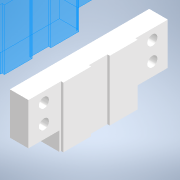
# Autodesk Inventor part: YCarriageBackHolder
Saved by Autodesk Inventor 2020 (Build 240168000, 168)
## iProperties
Created: 2022-04-26
Part Number: YCarriageBackHolder
Material: Tworzywo sztuczne ABS
Document SubType Name: Modeling
Designer: mikoma
Density: 1.06 g/cm^3
Appearance: Gładki — biały
Mass: 37.5008 g
Surface Area: 105.956 cm^2
Volume: 35.3781 cm^3
Author: mikoma
Autodesk Inventor part; units mm, degrees
ref_plane "YZ Plane" through (0, 0, 0) normal (1, 0, 0) x (0, 1, 0)
ref_plane "XZ Plane" through (0, 0, 0) normal (0, 1, 0) x (-1, 0, 0)
ref_plane "XY Plane" through (0, 0, 0) normal (0, 0, 1) x (1, 0, 0)
sketch "Szkic1" plane through (0, 0, 0) normal (0, 1, 0) x (-1, 0, 0)
  line L0 (12, 45) -> (0, 45)
  line L1 (0, 45) -> (0, -45)
  line L2 (0, -45) -> (12, -45)
  line L3 (12, -45) -> (12, 45)
  line L4 (0, 24) -> (-1.5, 24)
  line L5 (-1.5, 24) -> (-1.5, 6)
  line L6 (-1.5, 6) -> (0, 6)
  line L7 (0, 6) -> (0, 24)
  line L8 (0, -6) -> (-1.5, -6)
  line L9 (-1.5, -6) -> (-1.5, -24)
  line L10 (-1.5, -24) -> (0, -24)
  line L11 (0, -24) -> (0, -6)
  point P0 (0, 0)
  point P1 (0, -24)
  point P2 (0, 6)
  dimension "d0" = 90
  dimension "d1" = 12
  dimension "d2" = 45
  dimension "d3" = 21
  dimension "d4" = 18
  dimension "d5" = 1.5
  dimension "d6" = 21
  dimension "d7" = 18
  constraints: 24 end point, 6 parallel, 3 horizontal, 3 perpendicular, 2 point on line, 1 midpoint, 1 vertical alignment
  measures "d0" distance of L2.end L0.start
  measures "d1" distance of L1.end L2.end
  measures "d2" distance from line of L2 point (0, 0)
  measures "d3" distance between parallel lines of L0 L4
  measures "d4" distance between parallel lines of L4 L6
  measures "d5" distance from line of L0.end L5
  measures "d6" distance from line of L2 L9.end
  measures "d7" distance of L8.end L9.end
extrude "Wyciągnięcie proste1" add sketch "Szkic1" along normal blind 39
sketch "Szkic2" plane through (-12, 0, -45) normal (-1, 0, 0) x (0, 0, 1)
  circle A0 centre (10, 32.5) radius 3.25
  circle A1 centre (10, 20.5) radius 3.25
  circle A2 centre (80, 32.5) radius 3.25
  circle A3 centre (80, 20.5) radius 3.25
  line L0 (0, 39) -> (90, 39) projected
  line L1 (0, 0) -> (0, 39) projected
  line L2 (90, 0) -> (90, 39) projected
  line L3 (0, 0) -> (20, 0)
  line L4 (20, 0) -> (20, 12)
  line L5 (20, 12) -> (0, 12)
  line L6 (0, 12) -> (0, 0)
  line L7 (0, 0) -> (90, 0) projected
  line L8 (90, 0) -> (70, 0)
  line L9 (70, 0) -> (70, 12)
  line L10 (70, 12) -> (90, 12)
  line L11 (90, 12) -> (90, 0)
  line L12 (13.0311, 37.75) -> (16.0622, 32.5)
  line L13 (16.0622, 32.5) -> (13.0311, 27.25)
  line L14 (13.0311, 27.25) -> (6.9689, 27.25)
  line L15 (6.9689, 27.25) -> (3.9378, 32.5)
  line L16 (3.9378, 32.5) -> (6.9689, 37.75)
  line L17 (6.9689, 37.75) -> (13.0311, 37.75)
  line L18 (13.0311, 25.75) -> (16.0622, 20.5)
  line L19 (16.0622, 20.5) -> (13.0311, 15.25)
  line L20 (13.0311, 15.25) -> (6.9689, 15.25)
  line L21 (6.9689, 15.25) -> (3.9378, 20.5)
  line L22 (3.9378, 20.5) -> (6.9689, 25.75)
  line L23 (6.9689, 25.75) -> (13.0311, 25.75)
  line L24 (76.9689, 25.75) -> (83.0311, 25.75)
  line L25 (83.0311, 25.75) -> (86.0622, 20.5)
  line L26 (86.0622, 20.5) -> (83.0311, 15.25)
  line L27 (83.0311, 15.25) -> (76.9689, 15.25)
  line L28 (76.9689, 15.25) -> (73.9378, 20.5)
  line L29 (73.9378, 20.5) -> (76.9689, 25.75)
  line L30 (76.9689, 37.75) -> (83.0311, 37.75)
  line L31 (83.0311, 37.75) -> (86.0622, 32.5)
  line L32 (86.0622, 32.5) -> (83.0311, 27.25)
  line L33 (83.0311, 27.25) -> (76.9689, 27.25)
  line L34 (76.9689, 27.25) -> (73.9378, 32.5)
  line L35 (73.9378, 32.5) -> (76.9689, 37.75)
  point P0 (45, 0)
  point P1 (0, 12)
  dimension "d10" = 6.5
  dimension "d11" = 6.5
  dimension "d12" = 10
  dimension "d13" = 12
  dimension "d14" = 10
  dimension "d15" = 20
  dimension "d16" = 12
  dimension "d17" = 20
  dimension "d18" = 10.5
  dimension "d19" = 10.5
  dimension "d20" = 10.5
  dimension "d21" = 10.5
  constraints: 64 end point, 6 horizontal, 4 centre point, 4 coincident, 4 parallel, 3 equal radius, 3 horizontal alignment, 2 perpendicular, 2 vertical alignment, 52 other
  measures "d10" diameter of A0
  measures "d11" distance from line of L0 A0.centre
  measures "d12" distance from line of L1 A0.centre
  measures "d13" distance of A1.centre A0.centre
  measures "d14" distance from line of L2 A2.centre
  measures "d15" distance of L1.start L3.end
  measures "d16" distance of L3.end L4.end
  measures "d17" distance of L9.end L10.end
  measures "d18" distance between parallel lines of L14 L17
  measures "d19" distance between parallel lines of L20 L23
  measures "d20" distance between parallel lines of L33 L30
  measures "d21" distance between parallel lines of L27 L24
extrude "Wyciągnięcie proste2" cut sketch "Szkic2" against normal through all contours A0 | A1 | A2 | A3 | L5 L4 L3 L1 | L2 L7 L9 L10
extrude "Wyciągnięcie proste3" cut sketch "Szkic2" against normal blind 6 contours A0 | A1 | A2 | A3 | L12 L13 L14 L15 L16 L17 | L18 L19 L20 L21 L22 L23 | L24 L25 L26 L27 L28 L29 | L30 L31 L32 L33 L34 L35
equation "\"d14\" = d12"
equation "\"d19\" = d18"
equation "\"d20\" = d18"
equation "\"d21\" = d18"
